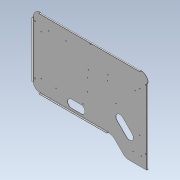
# Autodesk Inventor part: Монтажный лист
Saved by Autodesk Inventor 2021.2 (Build 252289000, 289)
## iProperties
Created: 2022-11-29
Part Number: Монтажный лист
Material: Типовые
Document SubType Name: ЛистМат
Designer: Voodoo
Density: 1 g/cm^3
Sheet Metal Rule: По умолчанию_мм
Appearance: По умолчанию
Mass: 115.884 g
Surface Area: 2338.39 cm^2
Volume: 115.884 cm^3
Author: Voodoo
Autodesk Inventor part; units mm, degrees
ref_plane "YZ Plane" through (0, 0, 0) normal (1, 0, 0) x (0, 1, 0)
ref_plane "XZ Plane" through (0, 0, 0) normal (0, 1, 0) x (-1, 0, 0)
ref_plane "XY Plane" through (0, 0, 0) normal (0, 0, 1) x (1, 0, 0)
sketch "Эскиз1" plane through (0, 0, 0) normal (0, 0, 1) x (1, 0, 0)
  line L0 (-186, -134.5) -> (65.5736, -134.5)
  line L1 (218, -134.5) -> (218, 102.5)
  line L2 (186, 134.5) -> (-186, 134.5)
  line L3 (-218, 102.5) -> (-218, -102.5)
  line L4 (-218, -134.5) -> (218, 134.5) construction
  line L5 (218, -134.5) -> (-218, 134.5) construction
  arc A0 (-186, 134.5) -> (-218, 102.5) centre (-186, 102.5) ccw
  arc A1 (218, 102.5) -> (186, 134.5) centre (186, 102.5) ccw
  arc A2 (-218, -102.5) -> (-186, -134.5) centre (-186, -102.5) ccw
  line L6 (218, -134.5) -> (218, -172.5)
  line L7 (206, -184.5) -> (140.4264, -184.5)
  line L8 (119.2132, -175.7132) -> (86.7868, -143.2868)
  arc A3 (206, -184.5) -> (218, -172.5) centre (206, -172.5) ccw
  arc A4 (119.2132, -175.7132) -> (140.4264, -184.5) centre (140.4264, -154.5) ccw
  arc A5 (86.7868, -143.2868) -> (65.5736, -134.5) centre (65.5736, -164.5) ccw
  line L9 (-186, 129.5) -> (186, 129.5)
  arc A6 (213, 102.5) -> (186, 129.5) centre (186, 102.5) ccw
  line L10 (213, 102.5) -> (213, -134.5)
  line L11 (213, -134.5) -> (213, -172.5)
  arc A7 (206, -179.5) -> (213, -172.5) centre (206, -172.5) ccw
  line L12 (206, -179.5) -> (140.4264, -179.5)
  arc A8 (122.7487, -172.1777) -> (140.4264, -179.5) centre (140.4264, -154.5) ccw
  line L13 (122.7487, -172.1777) -> (90.3223, -139.7513)
  arc A9 (90.3223, -139.7513) -> (65.5736, -129.5) centre (65.5736, -164.5) ccw
  line L14 (65.5736, -129.5) -> (-186, -129.5)
  arc A10 (-213, -102.5) -> (-186, -129.5) centre (-186, -102.5) ccw
  line L15 (-213, -102.5) -> (-213, 102.5)
  arc A11 (-186, 129.5) -> (-213, 102.5) centre (-186, 102.5) ccw
  point P0 (0, 0)
  point P1 (218, -184.5)
  point P2 (128, -184.5)
  dimension "d2" = 436
  dimension "d3" = 269
  dimension "d4" = 32
  dimension "d5" = 319
  dimension "d6" = 12
  dimension "d7" = 50
  dimension "d8" = 90
  dimension "d9" = 135
  dimension "d10" = 30
  dimension "d11" = 5
  constraints: 32 end point, 24 point on circle, 12 centre point, 12 point on line, 12 tangent, 4 parallel, 4 perpendicular, 3 equal radius, 2 midpoint, 1 horizontal, 12 other
  measures "d2" distance of L5.end L4.end
  measures "d3" distance of L4.end L1.start
  measures "d4" radius of A0
  measures "d5" distance between parallel lines of L7 L2
  measures "d6" radius of A3
  measures "d7" distance between parallel lines of L0 L7
  measures "d8" distance from line of L6 point (128, -184.5)
  measures "d9" angle of L0 L8
  measures "d10" radius of A4
  measures "d11" distance between parallel lines of L2 L9
extrude "Пластина1" add sketch "Эскиз1" along normal blind 1 contours L9 A6 L10 L11 A7 L12 A8 L13 A9 L14 A10 L15 A11
sketch "Эскиз4" plane through (-212, -102.5, 0) normal (-1, 0, 0) x (0, -1, 0)
  line L0 (-205, 0) -> (0, 0)
  line L1 (0, 0) -> (0, 6)
  line L2 (0, 6) -> (-205, 6)
  line L3 (-205, 6) -> (-205, 0)
  constraints: 6 end point, 1 horizontal, 1 perpendicular, 1 vertical
edge flange "Фланец1" height 6 angle 90 thickness 1 bend radius 1 thickness toward (-1, 0, 0) relief straight relief width 1 relief depth 0.5 corner gap 1 corner form 0 edges at (-213, 0, 1) (-60.2132, -129.5, 1) (0, 129.5, 1) (213, -16, 1) (213, -153.5, 1) wall of the first edge with corners at (-212, 102.5, 0) (-212, -102.5, 0) (-212, -102.5, 6) (-212, 102.5, 6)
bend "Сгиб1"
corner "УглСтык1"
sketch "Эскиз5" plane through (0, 0, 1) normal (0, 0, 1) x (1, 0, 0)
  arc A0 (-212.9815, -103.5) -> (-187, -129.4815) centre (-186, -102.5) ccw projected
  arc A1 (90.3223, -139.7513) -> (66.5736, -129.5143) centre (65.5736, -164.5) ccw projected
  line L0 (122.7487, -172.1777) -> (90.3223, -139.7513) projected
  arc A2 (122.7487, -172.1777) -> (140.4264, -179.5) centre (140.4264, -154.5) ccw projected
  line L1 (206, -179.5) -> (140.4264, -179.5) projected
  arc A3 (206, -179.5) -> (212.9282, -173.5) centre (206, -172.5) ccw projected
  arc A4 (212.9815, 103.5) -> (187, 129.4815) centre (186, 102.5) ccw projected
  arc A5 (-187, 129.4815) -> (-212.9815, 103.5) centre (-186, 102.5) ccw projected
  circle A6 centre (-204.9, 92.6) radius 2.5
  circle A7 centre (-204.9, -91.4) radius 2.5
  circle A8 centre (0, 121.6) radius 2.5
  circle A9 centre (205.1, 92.6) radius 2.5
  circle A10 centre (205.1, -128.4) radius 2.5
  line L2 (210.5, 103.5) -> (212.9815, 103.5) projected
  line L3 (187, 129.4815) -> (187, 127) projected
  line L4 (187, 127) -> (186, 127) projected
  line L5 (186, 127) -> (186, 127.5) projected
  line L6 (186, 127.5) -> (-186, 127.5) projected
  line L7 (-186, 127.5) -> (-186, 127) projected
  line L8 (-186, 127) -> (-187, 127) projected
  line L9 (-187, 127) -> (-187, 129.4815) projected
  line L10 (-212.9815, 103.5) -> (-210.5, 103.5) projected
  line L11 (-210.5, 103.5) -> (-210.5, 102.5) projected
  line L12 (-210.5, 102.5) -> (-211, 102.5) projected
  line L13 (-211, 102.5) -> (-211, -102.5) projected
  line L14 (-211, -102.5) -> (-210.5, -102.5) projected
  line L15 (-210.5, -102.5) -> (-210.5, -103.5) projected
  line L16 (-210.5, -103.5) -> (-212.9815, -103.5) projected
  line L17 (-187, -129.4815) -> (-187, -127) projected
  line L18 (-187, -127) -> (-186, -127) projected
  line L19 (-186, -127) -> (-186, -127.5) projected
  line L20 (-186, -127.5) -> (65.5736, -127.5) projected
  line L21 (65.5736, -127.5) -> (65.5736, -127) projected
  line L22 (65.5736, -127) -> (66.5736, -127) projected
  line L23 (66.5736, -127) -> (66.5736, -129.5143) projected
  line L24 (212.9282, -173.5) -> (210.5, -173.5) projected
  line L25 (210.5, -173.5) -> (210.5, -172.5) projected
  line L26 (210.5, -172.5) -> (211, -172.5) projected
  line L27 (211, -172.5) -> (211, 102.5) projected
  line L28 (211, 102.5) -> (210.5, 102.5) projected
  line L29 (210.5, 102.5) -> (210.5, 103.5) projected
  point P0 (0, 0)
  dimension "d34" = 5
  dimension "d37" = 5
  dimension "d38" = 184
  dimension "d40" = 5
  dimension "d43" = 5
  dimension "d45" = 5
  dimension "d47" = 51.1
  dimension "d48" = 221
  constraints: 5 centre point
  measures "d34" diameter of A6
  measures "d37" diameter of A7
  measures "d38" distance of A7.centre A6.centre
  measures "d40" diameter of A8
  measures "d43" diameter of A9
  measures "d45" diameter of A10
  measures "d47" distance from line of A10.centre L1
  measures "d48" distance of A10.centre A9.centre
extrude "Вырез3" cut sketch "Эскиз5" against normal blind 1 contours A6 | A7 | A8 | A9 | A10
sketch "Эскиз6" plane through (0, 0, 1) normal (0, 0, 1) x (1, 0, 0)
  circle A0 centre (205.1, 92.6) radius 2.5 projected
  circle A1 centre (-204.9, -91.4) radius 2.5 projected
  circle A2 centre (-204.9, 92.6) radius 2.5 projected
  circle A3 centre (0, 121.6) radius 2.5 projected
  circle A4 centre (205.1, -128.4) radius 2.5 projected
  arc A5 (-212.9815, -103.5) -> (-187, -129.4815) centre (-186, -102.5) ccw projected
  arc A6 (90.3223, -139.7513) -> (66.5736, -129.5143) centre (65.5736, -164.5) ccw projected
  line L0 (122.7487, -172.1777) -> (90.3223, -139.7513) projected
  arc A7 (122.7487, -172.1777) -> (140.4264, -179.5) centre (140.4264, -154.5) ccw projected
  line L1 (206, -179.5) -> (140.4264, -179.5) projected
  arc A8 (206, -179.5) -> (212.9282, -173.5) centre (206, -172.5) ccw projected
  arc A9 (212.9815, 103.5) -> (187, 129.4815) centre (186, 102.5) ccw projected
  arc A10 (-187, 129.4815) -> (-212.9815, 103.5) centre (-186, 102.5) ccw projected
  circle A11 centre (-8, 35) radius 1.5
  circle A12 centre (63, 35) radius 1.5
  circle A13 centre (64.5, 55) radius 1.5
  circle A14 centre (165.5, 55) radius 1.5
  circle A15 centre (-155.3, 86) radius 1.5
  circle A16 centre (-91, 86) radius 1.5
  line L2 (210.5, 103.5) -> (212.9815, 103.5) projected
  line L3 (187, 129.4815) -> (187, 127) projected
  line L4 (187, 127) -> (186, 127) projected
  line L5 (186, 127) -> (186, 127.5) projected
  line L6 (186, 127.5) -> (-186, 127.5) projected
  line L7 (-186, 127.5) -> (-186, 127) projected
  line L8 (-186, 127) -> (-187, 127) projected
  line L9 (-187, 127) -> (-187, 129.4815) projected
  line L10 (-212.9815, 103.5) -> (-210.5, 103.5) projected
  line L11 (-210.5, 103.5) -> (-210.5, 102.5) projected
  line L12 (-210.5, 102.5) -> (-211, 102.5) projected
  line L13 (-211, 102.5) -> (-211, -102.5) projected
  line L14 (-211, -102.5) -> (-210.5, -102.5) projected
  line L15 (-210.5, -102.5) -> (-210.5, -103.5) projected
  line L16 (-210.5, -103.5) -> (-212.9815, -103.5) projected
  line L17 (-187, -129.4815) -> (-187, -127) projected
  line L18 (-187, -127) -> (-186, -127) projected
  line L19 (-186, -127) -> (-186, -127.5) projected
  line L20 (-186, -127.5) -> (65.5736, -127.5) projected
  line L21 (65.5736, -127.5) -> (65.5736, -127) projected
  line L22 (65.5736, -127) -> (66.5736, -127) projected
  line L23 (66.5736, -127) -> (66.5736, -129.5143) projected
  line L24 (212.9282, -173.5) -> (210.5, -173.5) projected
  line L25 (210.5, -173.5) -> (210.5, -172.5) projected
  line L26 (210.5, -172.5) -> (211, -172.5) projected
  line L27 (211, -172.5) -> (211, 102.5) projected
  line L28 (211, 102.5) -> (210.5, 102.5) projected
  line L29 (210.5, 102.5) -> (210.5, 103.5) projected
  line L30 (-213, 102.5) -> (-213, -102.5) projected
  line L31 (186, 129.5) -> (-186, 129.5) projected
  line L32 (213, -172.5) -> (213, 102.5) projected
  point P0 (0, 0)
  dimension "d51" = 3
  dimension "d52" = 3
  dimension "d53" = 3
  dimension "d54" = 3
  dimension "d56" = 71
  dimension "d58" = 101
  dimension "d61" = 3
  dimension "d62" = 3
  dimension "d63" = 64.3
  dimension "d123" = 74.5
  dimension "d124" = 47.5
  dimension "d125" = 150
  dimension "d126" = 20
  dimension "d127" = 43.5
  dimension "d128" = 122
  constraints: 6 centre point, 3 horizontal alignment
  measures "d51" diameter of A11
  measures "d52" diameter of A12
  measures "d53" diameter of A13
  measures "d54" diameter of A14
  measures "d56" distance of A12.centre A11.centre
  measures "d58" distance of A13.centre A14.centre
  measures "d61" diameter of A15
  measures "d62" diameter of A16
  measures "d63" distance of A16.centre A15.centre
  measures "d123" distance from line of L31 A14.centre
  measures "d124" distance from line of L32 A14.centre
  measures "d125" distance from line of L32 A12.centre
  measures "d126" vertical distance of A13.centre A12.centre
  measures "d127" distance from line of A16.centre L31
  measures "d128" distance from line of L30 A16.centre
extrude "Вырез4" cut sketch "Эскиз6" against normal blind 1 contours A11 | A12 | A13 | A14 | A15 | A16
sketch "Эскиз7" plane through (0, 0, 1) normal (0, 0, 1) x (1, 0, 0)
  circle A0 centre (-155.3, 86) radius 1.5 projected
  circle A1 centre (64.5, 55) radius 1.5 projected
  circle A2 centre (-8, 35) radius 1.5 projected
  circle A3 centre (63, 35) radius 1.5 projected
  circle A4 centre (165.5, 55) radius 1.5 projected
  circle A5 centre (-91, 86) radius 1.5 projected
  circle A6 centre (205.1, 92.6) radius 2.5 projected
  circle A7 centre (-204.9, -91.4) radius 2.5 projected
  circle A8 centre (-204.9, 92.6) radius 2.5 projected
  circle A9 centre (0, 121.6) radius 2.5 projected
  circle A10 centre (205.1, -128.4) radius 2.5 projected
  arc A11 (-212.9815, -103.5) -> (-187, -129.4815) centre (-186, -102.5) ccw projected
  arc A12 (90.3223, -139.7513) -> (66.5736, -129.5143) centre (65.5736, -164.5) ccw projected
  line L0 (122.7487, -172.1777) -> (90.3223, -139.7513) projected
  arc A13 (122.7487, -172.1777) -> (140.4264, -179.5) centre (140.4264, -154.5) ccw projected
  line L1 (206, -179.5) -> (140.4264, -179.5) projected
  arc A14 (206, -179.5) -> (212.9282, -173.5) centre (206, -172.5) ccw projected
  arc A15 (212.9815, 103.5) -> (187, 129.4815) centre (186, 102.5) ccw projected
  arc A16 (-187, 129.4815) -> (-212.9815, 103.5) centre (-186, 102.5) ccw projected
  circle A17 centre (-182.5, 69.5) radius 1.5
  circle A18 centre (-182.5, -80.5) radius 1.5
  circle A19 centre (182.5, -80.5) radius 1.5
  circle A20 centre (182.5, 69.5) radius 1.5
  line L2 (0, 121.6) -> (0, 76.9707)
  line L3 (210.5, 103.5) -> (212.9815, 103.5) projected
  line L4 (187, 129.4815) -> (187, 127) projected
  line L5 (187, 127) -> (186, 127) projected
  line L6 (186, 127) -> (186, 127.5) projected
  line L7 (186, 127.5) -> (-186, 127.5) projected
  line L8 (-186, 127.5) -> (-186, 127) projected
  line L9 (-186, 127) -> (-187, 127) projected
  line L10 (-187, 127) -> (-187, 129.4815) projected
  line L11 (-212.9815, 103.5) -> (-210.5, 103.5) projected
  line L12 (-210.5, 103.5) -> (-210.5, 102.5) projected
  line L13 (-210.5, 102.5) -> (-211, 102.5) projected
  line L14 (-211, 102.5) -> (-211, -102.5) projected
  line L15 (-211, -102.5) -> (-210.5, -102.5) projected
  line L16 (-210.5, -102.5) -> (-210.5, -103.5) projected
  line L17 (-210.5, -103.5) -> (-212.9815, -103.5) projected
  line L18 (-187, -129.4815) -> (-187, -127) projected
  line L19 (-187, -127) -> (-186, -127) projected
  line L20 (-186, -127) -> (-186, -127.5) projected
  line L21 (-186, -127.5) -> (65.5736, -127.5) projected
  line L22 (65.5736, -127.5) -> (65.5736, -127) projected
  line L23 (65.5736, -127) -> (66.5736, -127) projected
  line L24 (66.5736, -127) -> (66.5736, -129.5143) projected
  line L25 (212.9282, -173.5) -> (210.5, -173.5) projected
  line L26 (210.5, -173.5) -> (210.5, -172.5) projected
  line L27 (210.5, -172.5) -> (211, -172.5) projected
  line L28 (211, -172.5) -> (211, 102.5) projected
  line L29 (211, 102.5) -> (210.5, 102.5) projected
  line L30 (210.5, 102.5) -> (210.5, 103.5) projected
  point P0 (0, 0)
  dimension "d68" = 3
  dimension "d69" = 3
  dimension "d70" = 3
  dimension "d71" = 3
  dimension "d72" = 182.5
  dimension "d74" = 150
  dimension "d75" = 365
  constraints: 4 centre point, 2 end point, 2 horizontal alignment, 2 vertical alignment, 1 vertical
  measures "d68" diameter of A17
  measures "d69" diameter of A18
  measures "d70" diameter of A19
  measures "d71" diameter of A20
  measures "d72" distance from line of A17.centre L2
  measures "d74" distance of A18.centre A17.centre
  measures "d75" distance of A17.centre A20.centre
extrude "Вырез5" cut sketch "Эскиз7" against normal blind 1 contours A17 | A18 | A19 | A20
sketch "Эскиз8" plane through (0, 0, 0) normal (0, 0, -1) x (-1, 0, 0)
  circle A0 centre (-182.5, -80.5) radius 1.5 projected
  circle A1 centre (182.5, 69.5) radius 1.5 projected
  circle A2 centre (182.5, -80.5) radius 1.5 projected
  circle A3 centre (-182.5, 69.5) radius 1.5 projected
  circle A4 centre (155.3, 86) radius 1.5 projected
  circle A5 centre (-64.5, 55) radius 1.5 projected
  circle A6 centre (8, 35) radius 1.5 projected
  circle A7 centre (-63, 35) radius 1.5 projected
  circle A8 centre (-165.5, 55) radius 1.5 projected
  circle A9 centre (91, 86) radius 1.5 projected
  circle A10 centre (-205.1, 92.6) radius 2.5 projected
  circle A11 centre (204.9, -91.4) radius 2.5 projected
  circle A12 centre (204.9, 92.6) radius 2.5 projected
  circle A13 centre (0, 121.6) radius 2.5 projected
  circle A14 centre (-205.1, -128.4) radius 2.5 projected
  line L0 (-212.9815, 103.5) -> (-210.5, 103.5) projected
  line L1 (-210.5, 103.5) -> (-210.5, 102.5) projected
  line L2 (-210.5, 102.5) -> (-211, 102.5) projected
  line L3 (-211, 102.5) -> (-211, -172.5) projected
  line L4 (-211, -172.5) -> (-210.5, -172.5) projected
  line L5 (-210.5, -172.5) -> (-210.5, -173.5) projected
  line L6 (-210.5, -173.5) -> (-212.9282, -173.5) projected
  arc A15 (-212.9282, -173.5) -> (-206, -179.5) centre (-206, -172.5) ccw projected
  line L7 (-206, -179.5) -> (-140.4264, -179.5) projected
  arc A16 (-140.4264, -179.5) -> (-122.7487, -172.1777) centre (-140.4264, -154.5) ccw projected
  line L8 (-122.7487, -172.1777) -> (-90.3223, -139.7513) projected
  arc A17 (-66.5736, -129.5143) -> (-90.3223, -139.7513) centre (-65.5736, -164.5) ccw projected
  line L9 (-66.5736, -129.5143) -> (-66.5736, -127) projected
  line L10 (-66.5736, -127) -> (-65.5736, -127) projected
  line L11 (-65.5736, -127) -> (-65.5736, -127.5) projected
  line L12 (-65.5736, -127.5) -> (186, -127.5) projected
  line L13 (186, -127.5) -> (186, -127) projected
  line L14 (186, -127) -> (187, -127) projected
  line L15 (187, -127) -> (187, -129.4815) projected
  arc A18 (187, -129.4815) -> (212.9815, -103.5) centre (186, -102.5) ccw projected
  line L16 (212.9815, -103.5) -> (210.5, -103.5) projected
  line L17 (210.5, -103.5) -> (210.5, -102.5) projected
  line L18 (210.5, -102.5) -> (211, -102.5) projected
  line L19 (211, -102.5) -> (211, 102.5) projected
  line L20 (211, 102.5) -> (210.5, 102.5) projected
  line L21 (210.5, 102.5) -> (210.5, 103.5) projected
  line L22 (210.5, 103.5) -> (212.9815, 103.5) projected
  arc A19 (212.9815, 103.5) -> (187, 129.4815) centre (186, 102.5) ccw projected
  line L23 (187, 129.4815) -> (187, 127) projected
  line L24 (187, 127) -> (186, 127) projected
  line L25 (186, 127) -> (186, 127.5) projected
  line L26 (186, 127.5) -> (-186, 127.5) projected
  line L27 (-186, 127.5) -> (-186, 127) projected
  line L28 (-186, 127) -> (-187, 127) projected
  line L29 (-187, 127) -> (-187, 129.4815) projected
  arc A20 (-187, 129.4815) -> (-212.9815, 103.5) centre (-186, 102.5) ccw projected
  line L30 (-108.5, -65) -> (-143.5, -100) construction
  line L31 (-119.1066, -54.3934) -> (-154.1066, -89.3934)
  line L32 (-132.8934, -110.6066) -> (-97.8934, -75.6066)
  arc A21 (-97.8934, -75.6066) -> (-119.1066, -54.3934) centre (-108.5, -65) ccw
  arc A22 (-154.1066, -89.3934) -> (-132.8934, -110.6066) centre (-143.5, -100) ccw
  point P0 (0, 0)
  point P1 (-126, -82.5)
  dimension "d80" = 30
  dimension "d81" = 45
  dimension "d82" = 45
  dimension "d83" = 85
  dimension "d84" = 35
  constraints: 8 end point, 4 point on circle, 4 tangent, 2 centre point, 1 midpoint, 1 parallel
  measures "d80" diameter of A22
  measures "d81" angle of L12 L30
  measures "d82" distance from line of L12 point (-126, -82.5)
  measures "d83" distance from line of L3 point (-126, -82.5)
  measures "d84" horizontal distance of L30.end L30.start
extrude "Вырез6" cut sketch "Эскиз8" against normal blind 1 contours A21 L32 A22 L31
sketch "Эскиз9" plane through (0, 0, 0) normal (0, 0, -1) x (-1, 0, 0)
  arc A0 (-154.1066, -89.3934) -> (-132.8934, -110.6066) centre (-143.5, -100) ccw projected
  line L0 (-154.1066, -89.3934) -> (-119.1066, -54.3934) projected
  arc A1 (-97.8934, -75.6066) -> (-119.1066, -54.3934) centre (-108.5, -65) ccw projected
  line L1 (-97.8934, -75.6066) -> (-132.8934, -110.6066) projected
  circle A2 centre (-182.5, -80.5) radius 1.5 projected
  circle A3 centre (182.5, 69.5) radius 1.5 projected
  circle A4 centre (182.5, -80.5) radius 1.5 projected
  circle A5 centre (-182.5, 69.5) radius 1.5 projected
  circle A6 centre (155.3, 86) radius 1.5 projected
  circle A7 centre (-64.5, 55) radius 1.5 projected
  circle A8 centre (8, 35) radius 1.5 projected
  circle A9 centre (-63, 35) radius 1.5 projected
  circle A10 centre (-165.5, 55) radius 1.5 projected
  circle A11 centre (91, 86) radius 1.5 projected
  circle A12 centre (-205.1, 92.6) radius 2.5 projected
  circle A13 centre (204.9, -91.4) radius 2.5 projected
  circle A14 centre (204.9, 92.6) radius 2.5 projected
  circle A15 centre (0, 121.6) radius 2.5 projected
  circle A16 centre (-205.1, -128.4) radius 2.5 projected
  line L2 (-212.9815, 103.5) -> (-210.5, 103.5) projected
  line L3 (-210.5, 103.5) -> (-210.5, 102.5) projected
  line L4 (-210.5, 102.5) -> (-211, 102.5) projected
  line L5 (-211, 102.5) -> (-211, -172.5) projected
  line L6 (-211, -172.5) -> (-210.5, -172.5) projected
  line L7 (-210.5, -172.5) -> (-210.5, -173.5) projected
  line L8 (-210.5, -173.5) -> (-212.9282, -173.5) projected
  arc A17 (-212.9282, -173.5) -> (-206, -179.5) centre (-206, -172.5) ccw projected
  line L9 (-206, -179.5) -> (-140.4264, -179.5) projected
  arc A18 (-140.4264, -179.5) -> (-122.7487, -172.1777) centre (-140.4264, -154.5) ccw projected
  line L10 (-122.7487, -172.1777) -> (-90.3223, -139.7513) projected
  arc A19 (-66.5736, -129.5143) -> (-90.3223, -139.7513) centre (-65.5736, -164.5) ccw projected
  line L11 (-66.5736, -129.5143) -> (-66.5736, -127) projected
  line L12 (-66.5736, -127) -> (-65.5736, -127) projected
  line L13 (-65.5736, -127) -> (-65.5736, -127.5) projected
  line L14 (-65.5736, -127.5) -> (186, -127.5) projected
  line L15 (186, -127.5) -> (186, -127) projected
  line L16 (186, -127) -> (187, -127) projected
  line L17 (187, -127) -> (187, -129.4815) projected
  arc A20 (187, -129.4815) -> (212.9815, -103.5) centre (186, -102.5) ccw projected
  line L18 (212.9815, -103.5) -> (210.5, -103.5) projected
  line L19 (210.5, -103.5) -> (210.5, -102.5) projected
  line L20 (210.5, -102.5) -> (211, -102.5) projected
  line L21 (211, -102.5) -> (211, 102.5) projected
  line L22 (211, 102.5) -> (210.5, 102.5) projected
  line L23 (210.5, 102.5) -> (210.5, 103.5) projected
  line L24 (210.5, 103.5) -> (212.9815, 103.5) projected
  arc A21 (212.9815, 103.5) -> (187, 129.4815) centre (186, 102.5) ccw projected
  line L25 (187, 129.4815) -> (187, 127) projected
  line L26 (187, 127) -> (186, 127) projected
  line L27 (186, 127) -> (186, 127.5) projected
  line L28 (186, 127.5) -> (-186, 127.5) projected
  line L29 (-186, 127.5) -> (-186, 127) projected
  line L30 (-186, 127) -> (-187, 127) projected
  line L31 (-187, 127) -> (-187, 129.4815) projected
  arc A22 (-187, 129.4815) -> (-212.9815, 103.5) centre (-186, 102.5) ccw projected
  circle A23 centre (-94, -22.5) radius 1.5
  circle A24 centre (11, -37.5) radius 1.5
  circle A25 centre (11, 7.5) radius 1.5
  point P0 (0, 0)
  dimension "d87" = 3
  dimension "d88" = 3
  dimension "d89" = 3
  dimension "d90" = 120
  dimension "d91" = 200
  dimension "d92" = 45
  dimension "d93" = 105
  dimension "d94" = 30
  constraints: 3 centre point, 1 vertical alignment
  measures "d87" diameter of A23
  measures "d88" diameter of A24
  measures "d89" diameter of A25
  measures "d90" distance from line of A25.centre L28
  measures "d91" distance from line of L21 A25.centre
  measures "d92" distance of A24.centre A25.centre
  measures "d93" horizontal distance of A25.centre A23.centre
  measures "d94" vertical distance of A23.centre A25.centre
extrude "Вырез7" cut sketch "Эскиз9" against normal blind 1 contours A23 | A24 | A25
sketch "Эскиз10" plane through (0, 0, 0) normal (0, 0, -1) x (-1, 0, 0)
  circle A0 centre (11, -37.5) radius 1.5 projected
  circle A1 centre (-94, -22.5) radius 1.5 projected
  circle A2 centre (11, 7.5) radius 1.5 projected
  arc A3 (-154.1066, -89.3934) -> (-132.8934, -110.6066) centre (-143.5, -100) ccw projected
  line L0 (-154.1066, -89.3934) -> (-119.1066, -54.3934) projected
  arc A4 (-97.8934, -75.6066) -> (-119.1066, -54.3934) centre (-108.5, -65) ccw projected
  line L1 (-97.8934, -75.6066) -> (-132.8934, -110.6066) projected
  circle A5 centre (-182.5, -80.5) radius 1.5 projected
  circle A6 centre (182.5, 69.5) radius 1.5 projected
  circle A7 centre (182.5, -80.5) radius 1.5 projected
  circle A8 centre (-182.5, 69.5) radius 1.5 projected
  circle A9 centre (155.3, 86) radius 1.5 projected
  circle A10 centre (-64.5, 55) radius 1.5 projected
  circle A11 centre (8, 35) radius 1.5 projected
  circle A12 centre (-63, 35) radius 1.5 projected
  circle A13 centre (-165.5, 55) radius 1.5 projected
  circle A14 centre (91, 86) radius 1.5 projected
  circle A15 centre (-205.1, 92.6) radius 2.5 projected
  circle A16 centre (204.9, -91.4) radius 2.5 projected
  circle A17 centre (204.9, 92.6) radius 2.5 projected
  circle A18 centre (0, 121.6) radius 2.5 projected
  circle A19 centre (-205.1, -128.4) radius 2.5 projected
  line L2 (-212.9815, 103.5) -> (-210.5, 103.5) projected
  line L3 (-210.5, 103.5) -> (-210.5, 102.5) projected
  line L4 (-210.5, 102.5) -> (-211, 102.5) projected
  line L5 (-211, 102.5) -> (-211, -172.5) projected
  line L6 (-211, -172.5) -> (-210.5, -172.5) projected
  line L7 (-210.5, -172.5) -> (-210.5, -173.5) projected
  line L8 (-210.5, -173.5) -> (-212.9282, -173.5) projected
  arc A20 (-212.9282, -173.5) -> (-206, -179.5) centre (-206, -172.5) ccw projected
  line L9 (-206, -179.5) -> (-140.4264, -179.5) projected
  arc A21 (-140.4264, -179.5) -> (-122.7487, -172.1777) centre (-140.4264, -154.5) ccw projected
  line L10 (-122.7487, -172.1777) -> (-90.3223, -139.7513) projected
  arc A22 (-66.5736, -129.5143) -> (-90.3223, -139.7513) centre (-65.5736, -164.5) ccw projected
  line L11 (-66.5736, -129.5143) -> (-66.5736, -127) projected
  line L12 (-66.5736, -127) -> (-65.5736, -127) projected
  line L13 (-65.5736, -127) -> (-65.5736, -127.5) projected
  line L14 (-65.5736, -127.5) -> (186, -127.5) projected
  line L15 (186, -127.5) -> (186, -127) projected
  line L16 (186, -127) -> (187, -127) projected
  line L17 (187, -127) -> (187, -129.4815) projected
  arc A23 (187, -129.4815) -> (212.9815, -103.5) centre (186, -102.5) ccw projected
  line L18 (212.9815, -103.5) -> (210.5, -103.5) projected
  line L19 (210.5, -103.5) -> (210.5, -102.5) projected
  line L20 (210.5, -102.5) -> (211, -102.5) projected
  line L21 (211, -102.5) -> (211, 102.5) projected
  line L22 (211, 102.5) -> (210.5, 102.5) projected
  line L23 (210.5, 102.5) -> (210.5, 103.5) projected
  line L24 (210.5, 103.5) -> (212.9815, 103.5) projected
  arc A24 (212.9815, 103.5) -> (187, 129.4815) centre (186, 102.5) ccw projected
  line L25 (187, 129.4815) -> (187, 127) projected
  line L26 (187, 127) -> (186, 127) projected
  line L27 (186, 127) -> (186, 127.5) projected
  line L28 (186, 127.5) -> (-186, 127.5) projected
  line L29 (-186, 127.5) -> (-186, 127) projected
  line L30 (-186, 127) -> (-187, 127) projected
  line L31 (-187, 127) -> (-187, 129.4815) projected
  arc A25 (-187, 129.4815) -> (-212.9815, 103.5) centre (-186, 102.5) ccw projected
  line L32 (35.5, -105.5) -> (70.5, -105.5) construction
  line L33 (35.5, -90.5) -> (70.5, -90.5)
  line L34 (70.5, -120.5) -> (35.5, -120.5)
  arc A26 (35.5, -90.5) -> (35.5, -120.5) centre (35.5, -105.5) ccw
  arc A27 (70.5, -120.5) -> (70.5, -90.5) centre (70.5, -105.5) ccw
  point P0 (0, 0)
  point P1 (53, -105.5)
  dimension "d97" = 7
  dimension "d98" = 35
  dimension "d99" = 30
  dimension "d100" = 158
  constraints: 8 end point, 4 point on circle, 4 tangent, 2 centre point, 1 horizontal, 1 midpoint, 1 parallel
  measures "d97" distance between parallel lines of L34 L14
  measures "d98" distance of L32.start L32.end
  measures "d99" distance between parallel lines of L34 L33
  measures "d100" distance from line of L21 point (53, -105.5)
extrude "Вырез8" cut sketch "Эскиз10" against normal blind 1 contours L33 A27 L34 A26
sketch "Эскиз11" plane through (0, 0, 0) normal (0, 0, -1) x (-1, 0, 0)
  arc A0 (35.5, -90.5) -> (35.5, -120.5) centre (35.5, -105.5) ccw projected
  line L0 (35.5, -90.5) -> (70.5, -90.5) projected
  arc A1 (70.5, -120.5) -> (70.5, -90.5) centre (70.5, -105.5) ccw projected
  line L1 (70.5, -120.5) -> (35.5, -120.5) projected
  circle A2 centre (11, -37.5) radius 1.5 projected
  circle A3 centre (-94, -22.5) radius 1.5 projected
  circle A4 centre (11, 7.5) radius 1.5 projected
  arc A5 (-154.1066, -89.3934) -> (-132.8934, -110.6066) centre (-143.5, -100) ccw projected
  line L2 (-154.1066, -89.3934) -> (-119.1066, -54.3934) projected
  arc A6 (-97.8934, -75.6066) -> (-119.1066, -54.3934) centre (-108.5, -65) ccw projected
  line L3 (-97.8934, -75.6066) -> (-132.8934, -110.6066) projected
  circle A7 centre (-182.5, -80.5) radius 1.5 projected
  circle A8 centre (182.5, 69.5) radius 1.5 projected
  circle A9 centre (182.5, -80.5) radius 1.5 projected
  circle A10 centre (-182.5, 69.5) radius 1.5 projected
  circle A11 centre (155.3, 86) radius 1.5 projected
  circle A12 centre (-64.5, 55) radius 1.5 projected
  circle A13 centre (8, 35) radius 1.5 projected
  circle A14 centre (-63, 35) radius 1.5 projected
  circle A15 centre (-165.5, 55) radius 1.5 projected
  circle A16 centre (91, 86) radius 1.5 projected
  circle A17 centre (-205.1, 92.6) radius 2.5 projected
  circle A18 centre (204.9, -91.4) radius 2.5 projected
  circle A19 centre (204.9, 92.6) radius 2.5 projected
  circle A20 centre (0, 121.6) radius 2.5 projected
  circle A21 centre (-205.1, -128.4) radius 2.5 projected
  line L4 (-212.9815, 103.5) -> (-210.5, 103.5) projected
  line L5 (-210.5, 103.5) -> (-210.5, 102.5) projected
  line L6 (-210.5, 102.5) -> (-211, 102.5) projected
  line L7 (-211, 102.5) -> (-211, -172.5) projected
  line L8 (-211, -172.5) -> (-210.5, -172.5) projected
  line L9 (-210.5, -172.5) -> (-210.5, -173.5) projected
  line L10 (-210.5, -173.5) -> (-212.9282, -173.5) projected
  arc A22 (-212.9282, -173.5) -> (-206, -179.5) centre (-206, -172.5) ccw projected
  line L11 (-206, -179.5) -> (-140.4264, -179.5) projected
  arc A23 (-140.4264, -179.5) -> (-122.7487, -172.1777) centre (-140.4264, -154.5) ccw projected
  line L12 (-122.7487, -172.1777) -> (-90.3223, -139.7513) projected
  arc A24 (-66.5736, -129.5143) -> (-90.3223, -139.7513) centre (-65.5736, -164.5) ccw projected
  line L13 (-66.5736, -129.5143) -> (-66.5736, -127) projected
  line L14 (-66.5736, -127) -> (-65.5736, -127) projected
  line L15 (-65.5736, -127) -> (-65.5736, -127.5) projected
  line L16 (-65.5736, -127.5) -> (186, -127.5) projected
  line L17 (186, -127.5) -> (186, -127) projected
  line L18 (186, -127) -> (187, -127) projected
  line L19 (187, -127) -> (187, -129.4815) projected
  arc A25 (187, -129.4815) -> (212.9815, -103.5) centre (186, -102.5) ccw projected
  line L20 (212.9815, -103.5) -> (210.5, -103.5) projected
  line L21 (210.5, -103.5) -> (210.5, -102.5) projected
  line L22 (210.5, -102.5) -> (211, -102.5) projected
  line L23 (211, -102.5) -> (211, 102.5) projected
  line L24 (211, 102.5) -> (210.5, 102.5) projected
  line L25 (210.5, 102.5) -> (210.5, 103.5) projected
  line L26 (210.5, 103.5) -> (212.9815, 103.5) projected
  arc A26 (212.9815, 103.5) -> (187, 129.4815) centre (186, 102.5) ccw projected
  line L27 (187, 129.4815) -> (187, 127) projected
  line L28 (187, 127) -> (186, 127) projected
  line L29 (186, 127) -> (186, 127.5) projected
  line L30 (186, 127.5) -> (-186, 127.5) projected
  line L31 (-186, 127.5) -> (-186, 127) projected
  line L32 (-186, 127) -> (-187, 127) projected
  line L33 (-187, 127) -> (-187, 129.4815) projected
  arc A27 (-187, 129.4815) -> (-212.9815, 103.5) centre (-186, 102.5) ccw projected
  circle A28 centre (28, -84.5) radius 1.5
  circle A29 centre (128, -84.5) radius 1.5
  line L34 (53, -90.5) -> (53, -99.1978) construction
  line L35 (186, -129.5) -> (-65.5736, -129.5) projected
  point P0 (0, 0)
  dimension "d114" = 3
  dimension "d115" = 3
  dimension "d116" = 25
  dimension "d117" = 75
  dimension "d118" = 45
  constraints: 2 centre point, 2 end point, 1 horizontal alignment, 1 midpoint, 1 vertical
  measures "d114" diameter of A28
  measures "d115" diameter of A29
  measures "d116" distance from line of A28.centre L34
  measures "d117" distance from line of L34 A29.centre
  measures "d118" distance from line of A28.centre L35
extrude "Вырез9" cut sketch "Эскиз11" against normal blind 1 contours A28 | A29
sketch "Эскиз13" plane through (0, 0, 0) normal (0, 0, -1) x (-1, 0, 0)
  circle A0 centre (28, -84.5) radius 1.5 projected
  circle A1 centre (128, -84.5) radius 1.5 projected
  arc A2 (35.5, -90.5) -> (35.5, -120.5) centre (35.5, -105.5) ccw projected
  line L0 (35.5, -90.5) -> (70.5, -90.5) projected
  arc A3 (70.5, -120.5) -> (70.5, -90.5) centre (70.5, -105.5) ccw projected
  line L1 (70.5, -120.5) -> (35.5, -120.5) projected
  circle A4 centre (11, -37.5) radius 1.5 projected
  circle A5 centre (-94, -22.5) radius 1.5 projected
  circle A6 centre (11, 7.5) radius 1.5 projected
  arc A7 (-154.1066, -89.3934) -> (-132.8934, -110.6066) centre (-143.5, -100) ccw projected
  line L2 (-154.1066, -89.3934) -> (-119.1066, -54.3934) projected
  arc A8 (-97.8934, -75.6066) -> (-119.1066, -54.3934) centre (-108.5, -65) ccw projected
  line L3 (-97.8934, -75.6066) -> (-132.8934, -110.6066) projected
  circle A9 centre (-182.5, -80.5) radius 1.5 projected
  circle A10 centre (182.5, 69.5) radius 1.5 projected
  circle A11 centre (182.5, -80.5) radius 1.5 projected
  circle A12 centre (-182.5, 69.5) radius 1.5 projected
  circle A13 centre (155.3, 86) radius 1.5 projected
  circle A14 centre (-64.5, 55) radius 1.5 projected
  circle A15 centre (8, 35) radius 1.5 projected
  circle A16 centre (-63, 35) radius 1.5 projected
  circle A17 centre (-165.5, 55) radius 1.5 projected
  circle A18 centre (91, 86) radius 1.5 projected
  circle A19 centre (-205.1, 92.6) radius 2.5 projected
  circle A20 centre (204.9, -91.4) radius 2.5 projected
  circle A21 centre (204.9, 92.6) radius 2.5 projected
  circle A22 centre (0, 121.6) radius 2.5 projected
  circle A23 centre (-205.1, -128.4) radius 2.5 projected
  line L4 (-212.9815, 103.5) -> (-210.5, 103.5) projected
  line L5 (-210.5, 103.5) -> (-210.5, 102.5) projected
  line L6 (-210.5, 102.5) -> (-211, 102.5) projected
  line L7 (-211, 102.5) -> (-211, -172.5) projected
  line L8 (-211, -172.5) -> (-210.5, -172.5) projected
  line L9 (-210.5, -172.5) -> (-210.5, -173.5) projected
  line L10 (-210.5, -173.5) -> (-212.9282, -173.5) projected
  arc A24 (-212.9282, -173.5) -> (-206, -179.5) centre (-206, -172.5) ccw projected
  line L11 (-206, -179.5) -> (-140.4264, -179.5) projected
  arc A25 (-140.4264, -179.5) -> (-122.7487, -172.1777) centre (-140.4264, -154.5) ccw projected
  line L12 (-122.7487, -172.1777) -> (-90.3223, -139.7513) projected
  arc A26 (-66.5736, -129.5143) -> (-90.3223, -139.7513) centre (-65.5736, -164.5) ccw projected
  line L13 (-66.5736, -129.5143) -> (-66.5736, -127) projected
  line L14 (-66.5736, -127) -> (-65.5736, -127) projected
  line L15 (-65.5736, -127) -> (-65.5736, -127.5) projected
  line L16 (-65.5736, -127.5) -> (186, -127.5) projected
  line L17 (186, -127.5) -> (186, -127) projected
  line L18 (186, -127) -> (187, -127) projected
  line L19 (187, -127) -> (187, -129.4815) projected
  arc A27 (187, -129.4815) -> (212.9815, -103.5) centre (186, -102.5) ccw projected
  line L20 (212.9815, -103.5) -> (210.5, -103.5) projected
  line L21 (210.5, -103.5) -> (210.5, -102.5) projected
  line L22 (210.5, -102.5) -> (211, -102.5) projected
  line L23 (211, -102.5) -> (211, 102.5) projected
  line L24 (211, 102.5) -> (210.5, 102.5) projected
  line L25 (210.5, 102.5) -> (210.5, 103.5) projected
  line L26 (210.5, 103.5) -> (212.9815, 103.5) projected
  arc A28 (212.9815, 103.5) -> (187, 129.4815) centre (186, 102.5) ccw projected
  line L27 (187, 129.4815) -> (187, 127) projected
  line L28 (187, 127) -> (186, 127) projected
  line L29 (186, 127) -> (186, 127.5) projected
  line L30 (186, 127.5) -> (-186, 127.5) projected
  line L31 (-186, 127.5) -> (-186, 127) projected
  line L32 (-186, 127) -> (-187, 127) projected
  line L33 (-187, 127) -> (-187, 129.4815) projected
  arc A29 (-187, 129.4815) -> (-212.9815, 103.5) centre (-186, 102.5) ccw projected
  circle A30 centre (-188, -144.5) radius 1.5
  circle A31 centre (-158, -144.5) radius 1.5
  line L34 (-213, -172.5) -> (-213, 102.5) projected
  point P0 (0, 0)
  dimension "d129" = 3
  dimension "d130" = 3
  dimension "d131" = 25
  dimension "d132" = 30
  dimension "d133" = 35
  constraints: 2 centre point, 1 horizontal alignment
  measures "d129" diameter of A30
  measures "d130" diameter of A31
  measures "d131" distance from line of A30.centre L34
  measures "d132" distance of A30.centre A31.centre
  measures "d133" distance from line of A30.centre L11
extrude "Вырез10" cut sketch "Эскиз13" against normal blind 1 contours A30 | A31
equation "\"d49\" = Толщина"
equation "\"d66\" = Толщина"
equation "\"d68\" = d69"
equation "\"d69\" = d70"
equation "\"d70\" = d71"
equation "\"d76\" = Толщина"
equation "\"d85\" = Толщина"
equation "\"d95\" = Толщина"
equation "\"d101\" = Толщина"
equation "\"d119\" = Толщина"
equation "\"d12\" = Толщина"
equation "\"d24\" = Ширина_просечки"
equation "\"d25\" = Глубина_просечки"
equation "\"d26\" = Мин_остаток"
equation "\"d27\" = Радиус_перехода"
equation "\"d30\" = Радиус_гибки"
equation "\"d31\" = Размер_просечки"
equation "\"d32\" = Размер_зазора"
equation "\"d33\" = Радиус_Якоби"
equation "\"Радиус_гибки\" = Толщина"
equation "\"Ширина_просечки\" = Толщина"
equation "\"Глубина_просечки\" = 0.5 * Толщина"
equation "\"Размер_просечки\" = 4 * Толщина"
equation "\"Мин_остаток\" = 2 * Толщина"
equation "\"Радиус_перехода\" = Радиус_гибки"
equation "\"Радиус_Якоби\" = Радиус_гибки"
equation "\"Размер_зазора\" = Толщина"
equation "\"Толщина\" = 1"
